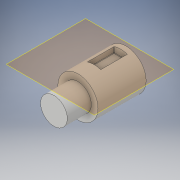
# Autodesk Inventor part: 軸1
Saved by Autodesk Inventor 2019.4 (Build 234330000, 330)
## iProperties
Created: 2019-12-29
Part Number: 軸1
Material: 一般
Document SubType Name: Modeling
Designer: Dorian Liu
Density: 1 g/cm^3
Appearance: 預設
Author: Dorian Liu
Autodesk Inventor part; units mm, degrees
ref_plane "YZ Plane" through (0, 0, 0) normal (1, 0, 0) x (0, 1, 0)
ref_plane "XY Plane" through (0, 0, 0) normal (0, 0, 1) x (1, 0, 0)
sketch "草圖2" plane through (0, 0, 0) normal (0, 0, 1) x (1, 0, 0)
  circle A0 centre (0, 0) radius 7.5
  dimension "d3" = 15
  constraints: 1 centre point, 1 coincident
  measures "d3" diameter of A0
extrude "擠出2" add sketch "草圖2" along normal blind 18
sketch "草圖3" plane through (0, 0, 18) normal (0, 0, 1) x (1, 0, 0)
  circle A0 centre (0, 0) radius 5
  dimension "d6" = 10
  constraints: 1 centre point, 1 coincident
  measures "d6" diameter of A0
extrude "擠出3" add sketch "草圖3" along normal blind 9
ref_plane "工作平面2" through (0, 7.5, 0) normal (0, 1, 0) x (-1, 0, 0)
sketch "草圖6" plane through (0, 7.5, 0) normal (0, 1, 0) x (-1, 0, 0)
  line L0 (-2.5, 12) -> (2.5, 12)
  line L1 (2.5, 12) -> (2.5, 2)
  line L2 (2.5, 2) -> (-2.5, 2)
  line L3 (-2.5, 2) -> (-2.5, 12)
  line L4 (-2.5, 12) -> (2.5, 2) construction
  line L5 (2.5, 12) -> (-2.5, 2) construction
  line L6 (-7.5, 0) -> (7.5, 0) projected
  point P0 (0, 0)
  point P1 (0, 7)
  dimension "d24" = 5
  dimension "d25" = 10
  dimension "d26" = 2
  dimension "d27" = 5
  constraints: 12 end point, 2 midpoint, 2 parallel, 1 horizontal, 1 perpendicular
  measures "d24" distance of L1.end L2.end
  measures "d25" distance of L0.end L1.end
  measures "d26" distance between parallel lines of L6 L2
  measures "d27" distance from line of L6.end L1
extrude "擠出6" cut sketch "草圖6" against normal blind 2.5
fillet "圓角3" radius 0.16 8 edges at (0, 5, 12) (2.5, 6.0355, 12) (2.5, 5, 7) (-2.5, 6.0355, 12) (-2.5, 5, 7) (-2.5, 6.0355, 2) (0, 5, 2) (2.5, 6.0355, 2)
